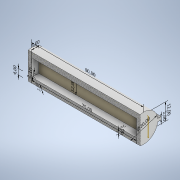
# Autodesk Inventor part: Inner_telescope_arm
Saved by Autodesk Inventor 2020 (Build 240168000, 168)
## iProperties
Created: 2019-08-27
Part Number: Inner_telescope_arm
Material: 常规
Document SubType Name: Modeling
Designer: User
Density: 1 g/cm^3
Appearance: 默认
Author: User
Autodesk Inventor part; units mm, degrees
sketch "草图1" plane through (0, 0, 0) normal (1, 0, 0) x (0, 1, 0)
  circle A0 centre (0, 0) radius 10
  dimension "d0" = 20
  constraints: 1 centre point, 1 coincident
  measures "d0" diameter of A0
extrude "拉伸1" add sketch "草图1" along normal blind 80
ref_plane "工作平面1" through (2.5, 0, 0) normal (1, 0, 0) x (0, 1, 0)
sketch "草图2" plane through (2.5, 0, 0) normal (1, 0, 0) x (0, 1, 0)
  circle A0 centre (0, 0) radius 10 projected
  line L0 (6, -2.4628) -> (-6, -2.4628)
  line L1 (-6, -2.4628) -> (-6, 2.5372)
  line L2 (-6, 2.5372) -> (6, 2.5372)
  line L3 (6, 2.5372) -> (6, -2.4628)
  line L4 (6.59, 0.0372) -> (-6.5609, 0.0372)
  point P0 (10, 0)
  point P1 (-10, 0)
  dimension "d4" = 4
  dimension "d5" = 4
  dimension "d6" = 5
  constraints: 10 end point, 3 horizontal, 2 parallel, 2 point on circle, 1 perpendicular, 1 other
  measures "d4" distance from line of A0.start L3
  measures "d5" distance from line of A0.end L1
  measures "d6" distance of L2.end L0.start
extrude "拉伸2" cut sketch "草图2" along normal blind 75 contours L0 L1 L4 L3 | L4 L1 L2 L3
ref_plane "工作平面3" through (0, 0, 10) normal (0, 0, 1) x (1, 0, 0)
sketch "草图5" plane through (0, 0, 10) normal (0, 0, 1) x (1, 0, 0)
  line L0 (-2.1953, 0) -> (98.9957, 0)
  line L1 (2.5, 6) -> (2.5, -6) projected
  line L2 (77.5, 6) -> (77.5, -6) projected
  line L3 (2.5, -6) -> (2.5, 6) projected
  line L4 (3.5, 4) -> (76.5, 4)
  line L5 (76.5, -4) -> (3.5, -4)
  line L6 (2.5, -3) -> (2.5, -2)
  arc A0 (3.5, 4) -> (3.5, 2) centre (3.5, 3) ccw
  arc A1 (3.5, -2) -> (3.5, -4) centre (3.5, -3) ccw
  line L7 (3.5, 2) -> (76.5, 2)
  line L8 (3.5, -2) -> (76.5, -2)
  arc A2 (76.5, 2) -> (76.5, 4) centre (76.5, 3) ccw
  circle A3 centre (76.5, -3) radius 1
  point P0 (0, 0)
  point P1 (3.5, 0)
  point P2 (76.5, 0)
  dimension "d52" = 8
  dimension "d53" = 1
  dimension "d54" = 1
  dimension "d55" = 1
  constraints: 12 end point, 9 point on circle, 4 centre point, 4 coincident, 4 horizontal, 4 tangent, 3 point on line, 1 parallel, 1 perpendicular, 1 other
  measures "d52" distance between parallel lines of L4 L5
  measures "d53" distance from line of point (3.5, 0) L1
  measures "d54" distance from line of L4 point (3.5, 3)
  measures "d55" distance from line of L5 point (3.5, -3)
extrude "拉伸3" cut sketch "草图5" against normal blind 7.5 contours A0 L4 A2 L7 | A1 L8 A3 L5
ref_plane "工作平面4" through (0, 0, -7) normal (0, 0, 1) x (1, 0, 0)
sketch "草图6" plane through (0, 0, -7) normal (0, 0, 1) x (1, 0, 0)
  line L0 (0, -10) -> (0, 10) projected
  line L1 (80, -10) -> (80, 10) projected
  line L2 (0, 1) -> (80, 1)
  line L3 (80, 1) -> (80, -1)
  line L4 (80, -1) -> (0, -1)
  line L5 (0, -1) -> (0, 1)
  line L6 (-22.5072, 0) -> (150.7978, 0)
  point P0 (0, 0)
  point P1 (0, -1)
  dimension "d39" = 2
  constraints: 10 end point, 3 parallel, 2 horizontal, 2 point on line, 1 perpendicular, 1 other
  measures "d39" distance between parallel lines of L4 L2
extrude "拉伸4" add sketch "草图6" against normal blind 5.5
ref_plane "工作平面5" through (2.5, -6, -2.4628) normal (0, 0, 1) x (1, 0, 0)
sketch "草图7" plane through (2.5, -6, -2.4628) normal (0, 0, 1) x (1, 0, 0)
  point P0 (-2.5, 6)
